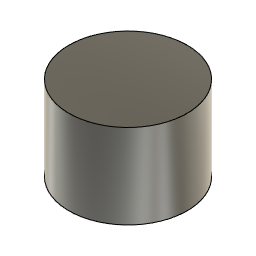
servo-arm v18 (Autodesk Fusion 360 archive; units mm, degrees)
design "knob-base"
Autodesk Fusion 360 part; units mm, degrees
sketch "Sketch1" plane through (0, 0, 0) normal (0, 0, 1) x (1, 0, 0)
  circle A0 centre (0, 0) radius 7
  dimension "d1" = 14
  constraint coincident A0.centre origin
  measures "d1" diameter of A0
extrude "Extrude1" add sketch "Sketch1" along normal blind 10

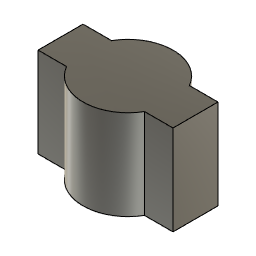
design "circular-knob"
Autodesk Fusion 360 part; units mm, degrees
sketch "Sketch1" plane through (0, 0, 0) normal (0, 0, 1) x (1, 0, 0)
  line L0 (-3.75, 1.25) -> (3.75, 1.25)
  line L1 (3.75, 1.25) -> (3.75, -1.25)
  line L2 (3.75, -1.25) -> (-3.75, -1.25)
  line L3 (-3.75, -1.25) -> (-3.75, 1.25)
  line L4 (-3.75, 1.25) -> (3.75, -1.25)
  line L5 (-3.75, -1.25) -> (3.75, 1.25)
  circle A0 centre (0, 0) radius 2.5
  dimension "d1" = 7.5
  dimension "d2" = 2.5
  dimension "d3" = 5
  constraint horizontal L0
  constraint vertical L1
  constraint horizontal L2
  constraint vertical L3
  constraint midpoint L4 A0.centre
  constraint coincident A0.centre origin
  measures "d1" distance of L0.start L0.end
  measures "d2" distance of L0.start L2.end
  measures "d3" diameter of A0
extrude "Extrude1" add sketch "Sketch1" along normal blind 5

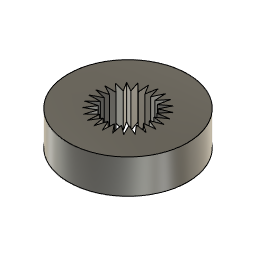
design "teeth-part"
Autodesk Fusion 360 part; units mm, degrees
sketch "Sketch15" plane through (0, 0, 0) normal (0, 0, 1) x (1, 0, 0)
  circle A0 centre (0, 0) radius 2.5
  circle A1 centre (0, 0) radius 7
  dimension "d65" = 5
  dimension "d67" = 14
  constraint coincident A0.centre A1.centre
  measures "d65" diameter of A0
  measures "d67" diameter of A1
extrude "Extrude12" add sketch "Sketch15" along normal blind 4 makes body 1
sketch "Sketch16" plane through (0, 0, 4) normal (0, 0, 1) x (-1, 0, 0)
  circle A0 centre (0, 0) radius 2.5
  circle A1 centre (0, 0) radius 7
  circle A2 centre (0, 0) radius 3.75
  line L0 (0, 0) -> (3.7204, 0.47)
  line L1 (0, 0) -> (3.75, 0) construction
  line L2 (0, 0) -> (3.7204, -0.47)
  line L3 (0, 0) -> (3.75, 0) construction
  line L4 (3.75, 0) -> (2.4803, -0.3133)
  line L5 (3.75, 0) -> (2.4803, 0.3133)
  dimension "d70" = 7.5
  dimension "d71" = 7.2
  dimension "d72" = 7.2
  constraint coincident A0.centre A1.centre
  constraint horizontal L1
  constraint horizontal L3
  constraint coincident L2 L4.end
  constraint coincident A0 L4.end
  constraint coincident L0 L5.end
  constraint coincident A0 L5.end
  measures "d70" diameter of A2
  measures "d71" angle of L0 L1
  measures "d72" angle of L2 L3
extrude "Extrude13" add sketch "Sketch16" against normal blind 4 separate body contours A0 L4 L5 makes body 2
pattern_circular "C-Pattern4" count 25 over 360 about axis through (0, 0, 1.75) along (0, 0, 1) of bodies 2 makes body 3 at (-3.2482, -0.7262, 2.6667) makes body 4 at (-2.9656, -1.5112, 2.6667) makes body 5 at (-2.3536, -2.3535, 2.6667) makes body 6 at (-1.6944, -2.8648, 2.6667) makes body 7 at (-0.9287, -3.1962, 2.6667) makes body 8 at (-0.1047, -3.3268, 2.6667) makes body 9 at (0.726, -3.2483, 2.6667) makes body 10 at (1.322, -3.0546, 2.6667) makes body 11 at (2.0401, -2.6299, 2.6667) makes body 12 at (2.63, -2.0399, 2.6667) makes body 13 at (3.1316, -1.1276, 2.6667) makes body 14 at (3.2874, -0.5206, 2.6667) makes body 15 at (3.2874, 0.5206, 2.6667) makes body 16 at (3.1316, 1.1276, 2.6667) makes body 17 at (2.63, 2.0399, 2.6667) makes body 18 at (2.0401, 2.6299, 2.6667) makes body 19 at (1.322, 3.0546, 2.6667) makes body 20 at (0.726, 3.2483, 2.6667) makes body 21 at (-0.3131, 3.3136, 2.6667) makes body 22 at (-1.1274, 3.1317, 2.6667) makes body 23 at (-1.8708, 2.7529, 2.6667) makes body 24 at (-2.4966, 2.2012, 2.6667) makes body 25 at (-2.9656, 1.5112, 2.6667) makes body 26 at (-3.2482, 0.7262, 2.6667)
combine "Combine4" operation cut target body 1 tool bodies 2 18 16 17 13 14 15 26 3 4 19 21 20 22 23 24 25 5 6 11 12 7 8 9 10
copy_body "Body->Comp1" bodies 1 removing the originals makes body 27 in component "Component"
component "Component" placed x (1, 0, 0) y (0, 1, 0) z (0, 0, 1) at (0, 0, 0)
